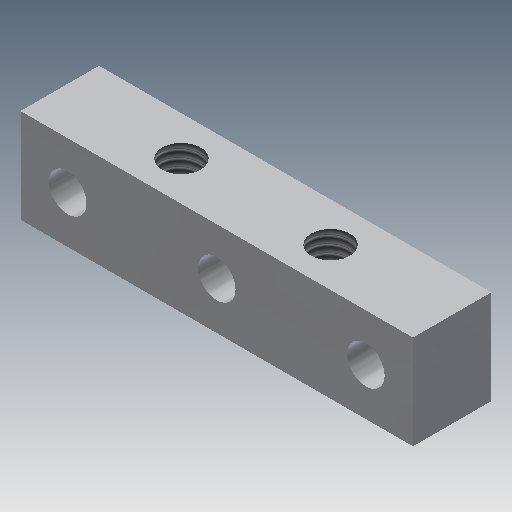
# Autodesk Inventor part: 足裏_サブフレーム_1_1
Saved by Autodesk Inventor 2017.3 (Build 213256000, 256)
## iProperties
Created: 2016-05-01
Part Number: 足裏_サブフレーム_1_1
Material: アルミニウム 2014-T4
Document SubType Name: Modeling
Designer: hiroaki
Density: 2.8 g/cm^3
Appearance: サテン
Mass: 1.75043 g
Surface Area: 7.6966 cm^2
Volume: 0.625153 cm^3
Author: hiroaki
Autodesk Inventor part; units mm, degrees
ref_plane "YZ Plane" through (0, 0, 0) normal (1, 0, 0) x (0, 1, 0)
ref_plane "XZ Plane" through (0, 0, 0) normal (0, 1, 0) x (-1, 0, 0)
ref_plane "XY Plane" through (0, 0, 0) normal (0, 0, 1) x (1, 0, 0)
derived "足裏_基礎_1.ipt"
sketch "スケッチ1" plane through (0, 0, 0) normal (0, 0, 1) x (1, 0, 0)
  circle A0 centre (0, 0) radius 5.05 construction
  line L0 (-21.25, 26.6) -> (21.25, 26.6) construction
  line L1 (21.25, 26.6) -> (21.25, -16) construction
  line L2 (21.25, -16) -> (-21.25, -16) construction
  line L3 (-21.25, -16) -> (-21.25, 26.6) construction
  circle A1 centre (0, 0) radius 26.6 construction
  line L4 (-12.5, -36) -> (12.5, -36) construction
  line L5 (12.5, -36) -> (12.5, -30) construction
  line L6 (12.5, -30) -> (10.9865, 0.5444) construction
  line L7 (-12.5, -36) -> (-12.5, -30) construction
  line L8 (-12.5, -30) -> (-10.9865, 0.5444) construction
  arc A2 (10.9865, 0.5444) -> (-10.9865, 0.5444) centre (0, 0) ccw construction
  line L9 (12.5, -30) -> (-12.5, -30) construction
  circle A3 centre (0, 8.5) radius 1.35 construction
  circle A4 centre (0, 8.5) radius 2.5 construction
  circle A5 centre (-8.5, 0) radius 1.35 construction
  circle A6 centre (0, -8.5) radius 1.35 construction
  circle A7 centre (8.5, 0) radius 1.35 construction
  circle A8 centre (-9.5, -33) radius 1.55 construction
  circle A9 centre (0, -33) radius 1.55 construction
  circle A10 centre (9.5, -33) radius 1.55 construction
  line L10 (-12.5, -33) -> (12.5, -33) construction
  line L11 (0, 0) -> (0, -30) construction
  line L12 (-12.5, -30) -> (12.5, -30)
  line L13 (12.5, -30) -> (12.5, -36)
  line L14 (12.5, -36) -> (-12.5, -36)
  line L15 (-12.5, -36) -> (-12.5, -30)
  circle A11 centre (-9.5, -33) radius 1.2
  circle A12 centre (0, -33) radius 1.2
  circle A13 centre (9.5, -33) radius 1.2
  line L16 (-6.3, -30) -> (-3.2, -30) construction
  line L17 (-3.2, -30) -> (-3.2, -36) construction
  line L18 (-3.2, -36) -> (-6.3, -36) construction
  line L19 (-6.3, -36) -> (-6.3, -30) construction
  line L20 (3.2, -30) -> (6.3, -30) construction
  line L21 (6.3, -30) -> (6.3, -36) construction
  line L22 (6.3, -36) -> (3.2, -36) construction
  line L23 (3.2, -36) -> (3.2, -30) construction
  line L24 (-4.75, -30) -> (-4.75, -36) construction
  line L25 (4.75, -30) -> (4.75, -36) construction
  point P0 (0, 26.6)
  point P1 (0, -36)
  dimension "d1" = 2.4
  dimension "d2" = 9.5
  dimension "d5" = 9.5
  measures "d1" diameter of A11
  measures "d2" distance of A9.centre A8.centre
  measures "d5" distance of A11.centre A12.centre
extrude "押し出し1" add sketch "スケッチ1" along normal blind 5
sketch "スケッチ3" plane through (-12.5, -30, 0) normal (0, 1, 0) x (1, 0, 0)
  line L0 (0, 0) -> (0, -5) projected
  line L1 (25, -5) -> (0, -5) projected
  line L2 (12.5, 0) -> (12.5, -5) construction
  point P0 (7.75, -2.5)
  point P1 (17.25, -2.5)
  point P2 (0, -2.5)
  dimension "d12" = 4.75
  constraints: 2 end point, 2 horizontal alignment, 2 midpoint, 1 symmetric about line
  measures "d12" distance from line of point (7.75, -2.5) L2
hole "穴1" at (-4.75, -30, 2.5) at (4.75, -30, 2.5) direction (0, -1, 0) diameter 2.459 end through all thread size "M3x0.5" class "6H" standard "ISO Metric profile"
equation "\"d5\" = d2"
equation "\"d12\" = 0.5 * d2"
